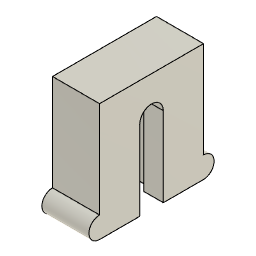
Piston (Autodesk Fusion 360 design; units mm, degrees)
Autodesk Fusion 360 part; units mm, degrees
note: some values were not read from the file. Set by a fixed rule: which sketch regions a step uses.
sketch "Boceto1" plane through (0, 0, 0) normal (0, 0, 1) x (1, 0, 0)
sketch "Boceto2" plane through (0, 0, 0) normal (1, 0, 0) x (0, 1, 0)
  line L0 (0, 0) -> (68.5, 0)
  line L1 (68.5, 0) -> (68.5, 77.5)
  line L2 (68.5, 77.5) -> (0, 77.5)
  line L3 (0, 77.5) -> (0, 0)
  line L4 (0, 0) -> (26.5, 0)
  line L5 (68.5, 0) -> (42, 0)
  line L6 (0, 0) -> (0, 7)
  line L7 (68.5, 0) -> (68.5, 7)
  circle A0 centre (0, 7) radius 7
  circle A1 centre (68.5, 7) radius 7
  line L8 (68.5, 14) -> (68.5, 52.5)
  line L9 (26.5, 0) -> (42, 0)
  line L10 (42, 0) -> (42, 52.5)
  line L11 (26.5, 52.5) -> (26.5, 0)
  circle A2 centre (34.25, 52.5) radius 7.75
  line L12 (26.5, 52.5) -> (26.5, 0)
  line L13 (42, 52.5) -> (42, 0)
  line L14 (26.5, 52.5) -> (42, 52.5)
  dimension "d2" = 77.5
  dimension "d3" = 26.5
  dimension "d4" = 26.5
  dimension "d9_1" = 15.5
  dimension "d89" = 68.5
  constraint horizontal L0
  constraint vertical L1
  constraint horizontal L2
  constraint vertical L3
  constraint coincident L0.start L3.end
  constraint perpendicular L3 L4
  constraint perpendicular L1 L5
  constraint perpendicular L0 L6
  constraint perpendicular L0 L7
  constraint coincident L6.end A0.centre
  constraint coincident L0.start A0
  constraint coincident L7.end A1.centre
  constraint coincident L0.end A1
  constraint coincident A1 L8.start
  constraint coincident L1 L8.start
  constraint parallel L1 L8
  constraint horizontal L9
  constraint vertical L10
  constraint vertical L11
  constraint perpendicular L9 L13
  constraint perpendicular L13 L14
  constraint midpoint A2.centre L14
  measures "d2" distance of L0.start L2.end
  measures "d3" distance of L0.start L4.end
  measures "d4" distance of L0.end L5.end
  measures "d9_1" diameter of A2
  measures "d89" distance of L1.end L2.end
sketch "Boceto3" plane through (0, 0, 0) normal (1, 0, 0) x (0, 1, 0)
extrude "Extruir2" add sketch "Boceto2" along normal blind 31 contours L0 L1 L2 L3 L4 L5 A0 A1 L8 L10 L11 A2 L12 L13 | L3 L6 A0 | L3 L6 A0 | L1 L7 A1 | L1 L7 A1
sketch "Boceto4" plane through (0, 26.5, 0) normal (0, 1, 0) x (-1, 0, 0)
  line L0 (0, 0) -> (0, 52.5)
  line L1 (0, 52.5) -> (-31, 52.5)
  line L2 (-31, 52.5) -> (-31, 0)
  line L3 (-31, 0) -> (0, 0)
  line L4 (-31, 0) -> (-21, 0)
  line L5 (-21, 0) -> (-13, 0)
  line L6 (-13, 0) -> (0, 0)
  dimension "d14_1" = 10
  dimension "d15_1" = 8
  constraint coincident L2.end L3.start
  constraint perpendicular L2 L4
  constraint parallel L3 L5
  constraint coincident L0.start L3.end
  measures "d14_1" distance of L2.end L4.end
  measures "d15_1" distance of L4.end L5.end
sketch "Boceto5" plane through (0, 0, 0) normal (0, 0, -1) x (1, 0, 0)
  line L0 (0, -42) -> (0, -68.5)
  line L1 (0, -68.5) -> (31, -68.5)
  line L2 (31, -68.5) -> (31, -42)
  line L3 (31, -42) -> (0, -42)
  line L4 (31, -42) -> (31, -26.5)
  line L5 (31, -26.5) -> (31, -34.25)
  line L6 (31, -34.25) -> (0, -34.25)
  line L7 (0, -34.25) -> (0, -22.05)
  line L8 (0, -34.25) -> (0, -46.45)
  line L9 (0, -34.25) -> (31, -34.25)
  line L10 (0, -34.25) -> (0, -22.05)
  line L11 (0, -22.05) -> (31, -22.05)
  line L12 (31, -22.05) -> (31, -34.25)
  line L13 (0, -46.45) -> (31, -46.45)
  line L14 (31, -46.45) -> (31, -22.05)
  line L15 (0, -22.05) -> (10, -22.05)
  line L16 (10, -22.05) -> (18.1, -22.05)
  line L17 (10, -22.05) -> (18.1, -22.05)
  line L18 (18.1, -22.05) -> (18.1, -46.45)
  line L19 (18.1, -46.45) -> (10, -46.45)
  line L20 (10, -46.45) -> (10, -22.05)
  dimension "d16_1" = 12.2
  dimension "d17_1" = 12.2
  dimension "d18_1" = 10
  dimension "d19" = 8.1
  dimension "d20" = 8.1
  constraint coincident L2.end L3.start
  constraint perpendicular L3 L4
  constraint midpoint L4 L5.end
  constraint perpendicular L4 L6
  constraint perpendicular L6 L7
  constraint perpendicular L6 L8
  constraint perpendicular L7 L11
  constraint perpendicular L6 L12
  constraint coincident L2 L13.end
  constraint perpendicular L2 L13
  constraint perpendicular L7 L15
  constraint parallel L11 L16
  constraint horizontal L17
  constraint vertical L18
  constraint horizontal L19
  constraint vertical L20
  measures "d16_1" distance of L6.end L7.end
  measures "d17_1" distance of L6.end L8.end
  measures "d18_1" distance of L7.end L15.end
  measures "d19" distance of L15.end L16.end
  measures "d20" distance of L15.end L16.end
extrude "Extruir3" cut sketch "Boceto5" against normal blind 52.5 contours L3 L6 L9 L18 L20 | L3 L13 L18 L19 L20 | L6 L9 L11 L16 L17 L18 L20
ref_plane "PlanoDeObra1" through (10, 44.225, 26.25) normal (1, 0, 0) x (0, 1, 0)
sketch "Boceto6" plane through (10, 44.975, 26.25) normal (1, 0, 0) x (0, 1, 0)
  circle A0 centre (-9.975, 26.25) radius 12.55
  dimension "d24_1" = 25.1
  measures "d24_1" diameter of A0
extrude "Extruir4" cut sketch "Boceto6" along normal blind 8.1
sketch "Boceto7" plane through (0, 0, 0) normal (0, 0, -1) x (1, 0, 0)
  line L0 (18.1, -22.05) -> (18.1, -26.5)
  line L1 (18.1, -26.5) -> (31, -26.5)
  line L2 (31, -26.5) -> (31, 0)
  line L3 (31, 0) -> (0, 0)
  line L4 (0, 0) -> (0, -26.5)
  line L5 (0, -26.5) -> (10, -26.5)
  line L6 (10, -26.5) -> (10, -22.05)
  line L7 (10, -22.05) -> (18.1, -22.05)
